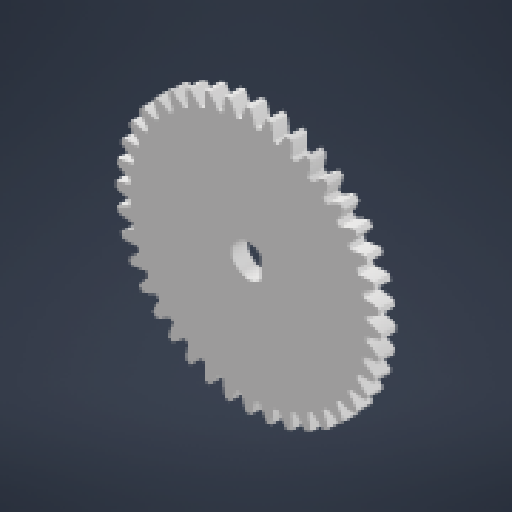
# Autodesk Inventor part: Central_axel_Gear
Saved by Autodesk Inventor 2026 (Build 300175050, 175E)
## iProperties
Created: 2026-04-30
Part Number: Central_axel_Gear
Material: Generic
Document SubType Name: Modeling
Designer: sniel
Density: 1 g/cm^3
Appearance: Default
Author: sniel
Autodesk Inventor part; units mm, degrees
ref_plane "YZ Plane" through (0, 0, 0) normal (1, 0, 0) x (0, 1, 0)
ref_plane "XZ Plane" through (0, 0, 0) normal (0, 1, 0) x (-1, 0, 0)
ref_plane "XY Plane" through (0, 0, 0) normal (0, 0, 1) x (1, 0, 0)
sketch "Sketch1" plane through (0, 0, 0) normal (0, 0, 1) x (1, 0, 0)
  arc A0 (-10.9505, -27.9782) -> (-11.02, -31.7791) centre (6.6967, -30.2023) ccw
  arc A1 (-11.02, -31.7791) -> (-9.7639, -32.1872) centre (0, 0) ccw
  arc A2 (-9.7639, -32.1872) -> (-7.5861, -29.0714) centre (-23.1702, -20.4979) ccw
  arc A3 (-7.5861, -29.0714) -> (-6.4389, -29.3468) centre (0, 0) ccw
  arc A4 (-6.4389, -29.3468) -> (-5.913, -33.1117) centre (11.3389, -28.7829) ccw
  arc A5 (-5.913, -33.1117) -> (-4.6085, -33.3184) centre (0, 0) ccw
  arc A6 (-4.6085, -33.3184) -> (-2.9449, -29.9002) centre (-19.6784, -23.8702) ccw
  arc A7 (-2.9449, -29.9002) -> (-1.7688, -29.9927) centre (0, 0) ccw
  arc A8 (-1.7688, -29.9927) -> (-0.6604, -33.6291) centre (15.702, -26.6547) ccw
  arc A9 (-0.6604, -33.6291) -> (0.6604, -33.6291) centre (0, 0) ccw
  arc A10 (0.6604, -33.6291) -> (1.7688, -29.9927) centre (-15.702, -26.6547) ccw
  arc A11 (1.7688, -29.9927) -> (2.9449, -29.9002) centre (0, 0) ccw
  arc A12 (2.9449, -29.9002) -> (4.6085, -33.3184) centre (19.6784, -23.8702) ccw
  arc A13 (4.6085, -33.3184) -> (5.913, -33.1117) centre (0, 0) ccw
  arc A14 (5.913, -33.1117) -> (6.4389, -29.3468) centre (-11.3389, -28.7829) ccw
  arc A15 (6.4389, -29.3468) -> (7.5861, -29.0714) centre (0, 0) ccw
  arc A16 (7.5861, -29.0714) -> (9.7639, -32.1872) centre (23.1702, -20.4979) ccw
  arc A17 (9.7639, -32.1872) -> (11.02, -31.7791) centre (0, 0) ccw
  arc A18 (11.02, -31.7791) -> (10.9505, -27.9782) centre (-6.6967, -30.2023) ccw
  arc A19 (10.9505, -27.9782) -> (12.0404, -27.5267) centre (0, 0) ccw
  arc A20 (12.0404, -27.5267) -> (14.6789, -30.2635) centre (26.0915, -16.621) ccw
  arc A21 (14.6789, -30.2635) -> (15.8557, -29.6639) centre (0, 0) ccw
  arc A22 (15.8557, -29.6639) -> (15.1924, -25.9207) centre (-1.8896, -30.878) ccw
  arc A23 (15.1924, -25.9207) -> (16.1983, -25.3043) centre (0, 0) ccw
  arc A24 (16.1983, -25.3043) -> (19.2324, -27.5947) centre (28.3704, -12.3347) ccw
  arc A25 (19.2324, -27.5947) -> (20.3009, -26.8183) centre (0, 0) ccw
  arc A26 (20.3009, -26.8183) -> (19.0602, -23.225) centre (2.9641, -30.7935) ccw
  arc A27 (19.0602, -23.225) -> (19.9574, -22.4588) centre (0, 0) ccw
  arc A28 (19.9574, -22.4588) -> (23.3124, -24.2463) centre (29.9507, -7.7447) ccw
  arc A29 (23.3124, -24.2463) -> (24.2463, -23.3124) centre (0, 0) ccw
  arc A30 (24.2463, -23.3124) -> (22.4588, -19.9574) centre (7.7447, -29.9507) ccw
  arc A31 (22.4588, -19.9574) -> (23.225, -19.0602) centre (0, 0) ccw
  arc A32 (23.225, -19.0602) -> (26.8183, -20.3009) centre (30.7935, -2.9641) ccw
  arc A33 (26.8183, -20.3009) -> (27.5947, -19.2324) centre (0, 0) ccw
  arc A34 (27.5947, -19.2324) -> (25.3043, -16.1983) centre (12.3347, -28.3704) ccw
  arc A35 (25.3043, -16.1983) -> (25.9207, -15.1924) centre (0, 0) ccw
  arc A36 (25.9207, -15.1924) -> (29.6639, -15.8557) centre (30.878, 1.8896) ccw
  arc A37 (29.6639, -15.8557) -> (30.2635, -14.6789) centre (0, 0) ccw
  arc A38 (30.2635, -14.6789) -> (27.5267, -12.0404) centre (16.621, -26.0915) ccw
  arc A39 (27.5267, -12.0404) -> (27.9782, -10.9505) centre (0, 0) ccw
  arc A40 (27.9782, -10.9505) -> (31.7791, -11.02) centre (30.2023, 6.6967) ccw
  arc A41 (31.7791, -11.02) -> (32.1872, -9.7639) centre (0, 0) ccw
  arc A42 (32.1872, -9.7639) -> (29.0714, -7.5861) centre (20.4979, -23.1702) ccw
  arc A43 (29.0714, -7.5861) -> (29.3468, -6.4389) centre (0, 0) ccw
  arc A44 (29.3468, -6.4389) -> (33.1117, -5.913) centre (28.7829, 11.3389) ccw
  arc A45 (33.1117, -5.913) -> (33.3184, -4.6085) centre (0, 0) ccw
  arc A46 (33.3184, -4.6085) -> (29.9002, -2.9449) centre (23.8702, -19.6784) ccw
  arc A47 (29.9002, -2.9449) -> (29.9927, -1.7688) centre (0, 0) ccw
  arc A48 (29.9927, -1.7688) -> (33.6291, -0.6604) centre (26.6547, 15.702) ccw
  arc A49 (33.6291, -0.6604) -> (33.6291, 0.6604) centre (0, 0) ccw
  arc A50 (33.6291, 0.6604) -> (29.9927, 1.7688) centre (26.6547, -15.702) ccw
  arc A51 (29.9927, 1.7688) -> (29.9002, 2.9449) centre (0, 0) ccw
  arc A52 (29.9002, 2.9449) -> (33.3184, 4.6085) centre (23.8702, 19.6784) ccw
  arc A53 (33.3184, 4.6085) -> (33.1117, 5.913) centre (0, 0) ccw
  arc A54 (33.1117, 5.913) -> (29.3468, 6.4389) centre (28.7829, -11.3389) ccw
  arc A55 (29.3468, 6.4389) -> (29.0714, 7.5861) centre (0, 0) ccw
  arc A56 (29.0714, 7.5861) -> (32.1872, 9.7639) centre (20.4979, 23.1702) ccw
  arc A57 (32.1872, 9.7639) -> (31.7791, 11.02) centre (0, 0) ccw
  arc A58 (31.7791, 11.02) -> (27.9782, 10.9505) centre (30.2023, -6.6967) ccw
  arc A59 (27.9782, 10.9505) -> (27.5267, 12.0404) centre (0, 0) ccw
  arc A60 (27.5267, 12.0404) -> (30.2635, 14.6789) centre (16.621, 26.0915) ccw
  arc A61 (30.2635, 14.6789) -> (29.6639, 15.8557) centre (0, 0) ccw
  arc A62 (29.6639, 15.8557) -> (25.9207, 15.1924) centre (30.878, -1.8896) ccw
  arc A63 (25.9207, 15.1924) -> (25.3043, 16.1983) centre (0, 0) ccw
  arc A64 (25.3043, 16.1983) -> (27.5947, 19.2324) centre (12.3347, 28.3704) ccw
  arc A65 (27.5947, 19.2324) -> (26.8183, 20.3009) centre (0, 0) ccw
  arc A66 (26.8183, 20.3009) -> (23.225, 19.0602) centre (30.7935, 2.9641) ccw
  arc A67 (23.225, 19.0602) -> (22.4588, 19.9574) centre (0, 0) ccw
  arc A68 (22.4588, 19.9574) -> (24.2463, 23.3124) centre (7.7447, 29.9507) ccw
  arc A69 (24.2463, 23.3124) -> (23.3124, 24.2463) centre (0, 0) ccw
  arc A70 (23.3124, 24.2463) -> (19.9574, 22.4588) centre (29.9507, 7.7447) ccw
  arc A71 (19.9574, 22.4588) -> (19.0602, 23.225) centre (0, 0) ccw
  arc A72 (19.0602, 23.225) -> (20.3009, 26.8183) centre (2.9641, 30.7935) ccw
  arc A73 (20.3009, 26.8183) -> (19.2324, 27.5947) centre (0, 0) ccw
  arc A74 (19.2324, 27.5947) -> (16.1983, 25.3043) centre (28.3704, 12.3347) ccw
  arc A75 (16.1983, 25.3043) -> (15.1924, 25.9207) centre (0, 0) ccw
  arc A76 (15.1924, 25.9207) -> (15.8557, 29.6639) centre (-1.8896, 30.878) ccw
  arc A77 (15.8557, 29.6639) -> (14.6789, 30.2635) centre (0, 0) ccw
  arc A78 (14.6789, 30.2635) -> (12.0404, 27.5267) centre (26.0915, 16.621) ccw
  arc A79 (12.0404, 27.5267) -> (10.9505, 27.9782) centre (0, 0) ccw
  arc A80 (10.9505, 27.9782) -> (11.02, 31.7791) centre (-6.6967, 30.2023) ccw
  arc A81 (11.02, 31.7791) -> (9.7639, 32.1872) centre (0, 0) ccw
  arc A82 (9.7639, 32.1872) -> (7.5861, 29.0714) centre (23.1702, 20.4979) ccw
  arc A83 (7.5861, 29.0714) -> (6.4389, 29.3468) centre (0, 0) ccw
  arc A84 (6.4389, 29.3468) -> (5.913, 33.1117) centre (-11.3389, 28.7829) ccw
  arc A85 (5.913, 33.1117) -> (4.6085, 33.3184) centre (0, 0) ccw
  arc A86 (4.6085, 33.3184) -> (2.9449, 29.9002) centre (19.6784, 23.8702) ccw
  arc A87 (2.9449, 29.9002) -> (1.7688, 29.9927) centre (0, 0) ccw
  arc A88 (1.7688, 29.9927) -> (0.6604, 33.6291) centre (-15.702, 26.6547) ccw
  arc A89 (0.6604, 33.6291) -> (-0.6604, 33.6291) centre (0, 0) ccw
  arc A90 (-0.6604, 33.6291) -> (-1.7688, 29.9927) centre (15.702, 26.6547) ccw
  arc A91 (-1.7688, 29.9927) -> (-2.9449, 29.9002) centre (0, 0) ccw
  arc A92 (-2.9449, 29.9002) -> (-4.6085, 33.3184) centre (-19.6784, 23.8702) ccw
  arc A93 (-4.6085, 33.3184) -> (-5.913, 33.1117) centre (0, 0) ccw
  arc A94 (-5.913, 33.1117) -> (-6.4389, 29.3468) centre (11.3389, 28.7829) ccw
  arc A95 (-6.4389, 29.3468) -> (-7.5861, 29.0714) centre (0, 0) ccw
  arc A96 (-7.5861, 29.0714) -> (-9.7639, 32.1872) centre (-23.1702, 20.4979) ccw
  arc A97 (-9.7639, 32.1872) -> (-11.02, 31.7791) centre (0, 0) ccw
  arc A98 (-11.02, 31.7791) -> (-10.9505, 27.9782) centre (6.6967, 30.2023) ccw
  arc A99 (-10.9505, 27.9782) -> (-12.0404, 27.5267) centre (0, 0) ccw
  arc A100 (-12.0404, 27.5267) -> (-14.6789, 30.2635) centre (-26.0915, 16.621) ccw
  arc A101 (-14.6789, 30.2635) -> (-15.8557, 29.6639) centre (0, 0) ccw
  arc A102 (-15.8557, 29.6639) -> (-15.1924, 25.9207) centre (1.8896, 30.878) ccw
  arc A103 (-15.1924, 25.9207) -> (-16.1983, 25.3043) centre (0, 0) ccw
  arc A104 (-16.1983, 25.3043) -> (-19.2324, 27.5947) centre (-28.3704, 12.3347) ccw
  arc A105 (-19.2324, 27.5947) -> (-20.3009, 26.8183) centre (0, 0) ccw
  arc A106 (-20.3009, 26.8183) -> (-19.0602, 23.225) centre (-2.9641, 30.7935) ccw
  arc A107 (-19.0602, 23.225) -> (-19.9574, 22.4588) centre (0, 0) ccw
  arc A108 (-19.9574, 22.4588) -> (-23.3124, 24.2463) centre (-29.9507, 7.7447) ccw
  arc A109 (-23.3124, 24.2463) -> (-24.2463, 23.3124) centre (0, 0) ccw
  arc A110 (-24.2463, 23.3124) -> (-22.4588, 19.9574) centre (-7.7447, 29.9507) ccw
  arc A111 (-22.4588, 19.9574) -> (-23.225, 19.0602) centre (0, 0) ccw
  arc A112 (-23.225, 19.0602) -> (-26.8183, 20.3009) centre (-30.7935, 2.9641) ccw
  arc A113 (-26.8183, 20.3009) -> (-27.5947, 19.2324) centre (0, 0) ccw
  arc A114 (-27.5947, 19.2324) -> (-25.3043, 16.1983) centre (-12.3347, 28.3704) ccw
  arc A115 (-25.3043, 16.1983) -> (-25.9207, 15.1924) centre (0, 0) ccw
  arc A116 (-25.9207, 15.1924) -> (-29.6639, 15.8557) centre (-30.878, -1.8896) ccw
  arc A117 (-29.6639, 15.8557) -> (-30.2635, 14.6789) centre (0, 0) ccw
  arc A118 (-30.2635, 14.6789) -> (-27.5267, 12.0404) centre (-16.621, 26.0915) ccw
  arc A119 (-27.5267, 12.0404) -> (-27.9782, 10.9505) centre (0, 0) ccw
  arc A120 (-27.9782, 10.9505) -> (-31.7791, 11.02) centre (-30.2023, -6.6967) ccw
  arc A121 (-31.7791, 11.02) -> (-32.1872, 9.7639) centre (0, 0) ccw
  arc A122 (-32.1872, 9.7639) -> (-29.0714, 7.5861) centre (-20.4979, 23.1702) ccw
  arc A123 (-29.0714, 7.5861) -> (-29.3468, 6.4389) centre (0, 0) ccw
  arc A124 (-29.3468, 6.4389) -> (-33.1117, 5.913) centre (-28.7829, -11.3389) ccw
  arc A125 (-33.1117, 5.913) -> (-33.3184, 4.6085) centre (0, 0) ccw
  arc A126 (-33.3184, 4.6085) -> (-29.9002, 2.9449) centre (-23.8702, 19.6784) ccw
  arc A127 (-29.9002, 2.9449) -> (-29.9927, 1.7688) centre (0, 0) ccw
  arc A128 (-29.9927, 1.7688) -> (-33.6291, 0.6604) centre (-26.6547, -15.702) ccw
  arc A129 (-33.6291, 0.6604) -> (-33.6291, -0.6604) centre (0, 0) ccw
  arc A130 (-33.6291, -0.6604) -> (-29.9927, -1.7688) centre (-26.6547, 15.702) ccw
  arc A131 (-29.9927, -1.7688) -> (-29.9002, -2.9449) centre (0, 0) ccw
  arc A132 (-29.9002, -2.9449) -> (-33.3184, -4.6085) centre (-23.8702, -19.6784) ccw
  arc A133 (-33.3184, -4.6085) -> (-33.1117, -5.913) centre (0, 0) ccw
  arc A134 (-33.1117, -5.913) -> (-29.3468, -6.4389) centre (-28.7829, 11.3389) ccw
  arc A135 (-29.3468, -6.4389) -> (-29.0714, -7.5861) centre (0, 0) ccw
  arc A136 (-29.0714, -7.5861) -> (-32.1872, -9.7639) centre (-20.4979, -23.1702) ccw
  arc A137 (-32.1872, -9.7639) -> (-31.7791, -11.02) centre (0, 0) ccw
  arc A138 (-31.7791, -11.02) -> (-27.9782, -10.9505) centre (-30.2023, 6.6967) ccw
  arc A139 (-27.9782, -10.9505) -> (-27.5267, -12.0404) centre (0, 0) ccw
  arc A140 (-27.5267, -12.0404) -> (-30.2635, -14.6789) centre (-16.621, -26.0915) ccw
  arc A141 (-30.2635, -14.6789) -> (-29.6639, -15.8557) centre (0, 0) ccw
  arc A142 (-29.6639, -15.8557) -> (-25.9207, -15.1924) centre (-30.878, 1.8896) ccw
  arc A143 (-25.9207, -15.1924) -> (-25.3043, -16.1983) centre (0, 0) ccw
  arc A144 (-25.3043, -16.1983) -> (-27.5947, -19.2324) centre (-12.3347, -28.3704) ccw
  arc A145 (-27.5947, -19.2324) -> (-26.8183, -20.3009) centre (0, 0) ccw
  arc A146 (-26.8183, -20.3009) -> (-23.225, -19.0602) centre (-30.7935, -2.9641) ccw
  arc A147 (-23.225, -19.0602) -> (-22.4588, -19.9574) centre (0, 0) ccw
  arc A148 (-22.4588, -19.9574) -> (-24.2463, -23.3124) centre (-7.7447, -29.9507) ccw
  arc A149 (-24.2463, -23.3124) -> (-23.3124, -24.2463) centre (0, 0) ccw
  arc A150 (-23.3124, -24.2463) -> (-19.9574, -22.4588) centre (-29.9507, -7.7447) ccw
  arc A151 (-19.9574, -22.4588) -> (-19.0602, -23.225) centre (0, 0) ccw
  arc A152 (-19.0602, -23.225) -> (-20.3009, -26.8183) centre (-2.9641, -30.7935) ccw
  arc A153 (-20.3009, -26.8183) -> (-19.2324, -27.5947) centre (0, 0) ccw
  arc A154 (-19.2324, -27.5947) -> (-16.1983, -25.3043) centre (-28.3704, -12.3347) ccw
  arc A155 (-16.1983, -25.3043) -> (-15.1924, -25.9207) centre (0, 0) ccw
  arc A156 (-15.1924, -25.9207) -> (-15.8557, -29.6639) centre (1.8896, -30.878) ccw
  arc A157 (-15.8557, -29.6639) -> (-14.6789, -30.2635) centre (0, 0) ccw
  arc A158 (-14.6789, -30.2635) -> (-12.0404, -27.5267) centre (-26.0915, -16.621) ccw
  arc A159 (-12.0404, -27.5267) -> (-10.9505, -27.9782) centre (0, 0) ccw
  circle A160 centre (0, 0) radius 4.1
  line L0 (0, 0) -> (4.1, 0)
  line L1 (4.1, 0) -> (3.1, 0)
  line L2 (3.1, 0) -> (3.1, -2.6833)
  line L3 (3.1, 0) -> (3.1, 2.6833)
  point P0 (0, 0)
  point P1 (2.1, -3.5214)
  point P2 (2.1, 3.5214)
  dimension "d2" = 8.2
  dimension "d4" = 1
  constraints: 325 point on circle, 161 centre point, 8 end point, 2 point on line, 1 coincident, 1 horizontal, 1 perpendicular
  measures "d2" diameter of A160
  measures "d4" distance of L0.end L1.end
extrude "Extrusion1" add sketch "Sketch1" along normal blind 4 contours A159 A158 A157 A156 A155 A154 A153 A152 A151 A150 A149 A148 A147 A146 A145 A144 A143 A142 A141 A140 A139 A138 A137 A136 A135 A134 A133 A132 A131 A130 A129 A128 A127 A126 A125 A124 A123 A122 A121 A120 A119 A118 A117 A116 A115 A114 A113 A112 A111 A110 A109 A108 A107 A106 A105 A104 A103 A102 A101 A100 A99 A98 A97 A96 A95 A94 A93 A92 A91 A90 A89 A88 A87 A86 A85 A84 A83 A82 A81 A80 A79 A78 A77 A76 A75 A74 A73 A72 A71 A70 A69 A68 A67 A66 A65 A64 A63 A62 A61 A60 A59 A58 A57 A56 A55 A54 A53 A52 A51 A50 A49 A48 A47 A46 A45 A44 A43 A42 A41 A40 A39 A38 A37 A36 A35 A34 A33 A32 A31 A30 A29 A28 A27 A26 A25 A24 A23 A22 A21 A20 A19 A18 A17 A16 A15 A14 A13 A12 A11 A10 A9 A8 A7 A6 A5 A4 A3 A2 A1 A0 | L0 L3 A160 | A160 L2 L0
body "Solid1"
